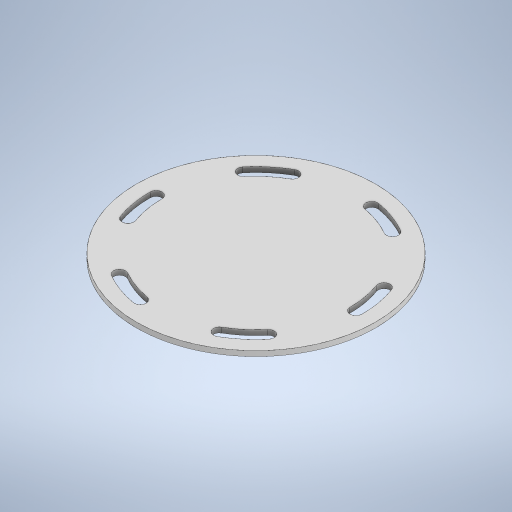
# Autodesk Inventor part: Bottom_plate
Saved by Autodesk Inventor 2024.3 (Build 283343000, 343)
## iProperties
Created: 2025-03-09
Part Number: Bottom_plate
Material: Generic
Document SubType Name: Modeling
Designer: ajclo
Density: 1 g/cm^3
Appearance: Default
Author: ajclo
Autodesk Inventor part; units mm, degrees
ref_plane "YZ Plane" through (0, 0, 0) normal (1, 0, 0) x (0, 1, 0)
ref_plane "XZ Plane" through (0, 0, 0) normal (0, 1, 0) x (-1, 0, 0)
ref_plane "XY Plane" through (0, 0, 0) normal (0, 0, 1) x (1, 0, 0)
sketch "Sketch1" plane through (0, 0, 0) normal (0, 1, 0) x (-1, 0, 0)
  circle A0 centre (0, 0) radius 70
  dimension "d0" = 140
  constraints: 1 centre point, 1 coincident
  measures "d0" diameter of A0
extrude "Extrusion1" add sketch "Sketch1" along normal blind 3
sketch "Sketch2" plane through (0, 3, 0) normal (0, 1, 0) x (1, 0, 0)
  circle A0 centre (0, 0) radius 62
  circle A1 centre (0, 0) radius 55
  arc A2 (-55, 0) -> (-62, 0) centre (-58.5, 0) ccw
  arc A3 (-58.2641, -21.1966) -> (-51.6859, -18.8034) centre (-54.975, -20) ccw
  dimension "d3" = 124
  dimension "d4" = 110
  dimension "d7" = 20
  constraints: 8 point on circle, 4 centre point, 4 tangent, 2 coincident
  measures "d3" diameter of A0
  measures "d4" diameter of A1
  measures "d7" vertical distance of point (0, 0) A3.centre
extrude "Extrusion2" cut sketch "Sketch2" against normal through all contours A2 A1 A3 A0 picked at (-56.7601, -18.0974)
pattern_circular "Circular Pattern1" count 6 over 360 about axis through (0, 0, 0) along (0, 1, 0) of "Extrusion2"
body "Solid1"
